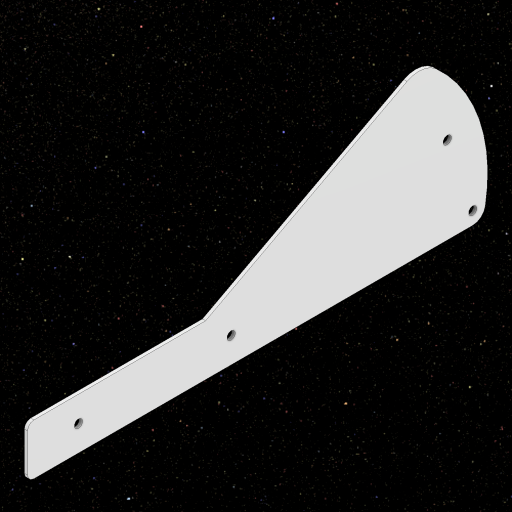
# Autodesk Inventor part: gusset_no_motor
Saved by Autodesk Inventor 2024 (Build 280153000, 153)
## iProperties
Created: 2024-02-12
Part Number: gusset_no_motor
Material: Acetal Resin, White
Document SubType Name: Modeling
Designer: Averey Ku
Density: 1.425 g/cm^3
Appearance: Smooth - White
Author: Averey Ku
Autodesk Inventor part; units mm, degrees
ref_plane "YZ Plane" through (0, 0, 0) normal (1, 0, 0) x (0, 1, 0)
ref_plane "XZ Plane" through (0, 0, 0) normal (0, 1, 0) x (-1, 0, 0)
ref_plane "XY Plane" through (0, 0, 0) normal (0, 0, 1) x (1, 0, 0)
sketch "main" plane through (0, 0, 0) normal (0, 0, 1) x (1, 0, 0)
  circle A0 centre (-31.9195, -99.4713) radius 2.0955
  arc A1 (-38.2695, -99.4713) -> (-33.0376, -105.722) centre (-31.9195, -99.4713) ccw
  arc A2 (-33.0376, -105.722) -> (38.5686, -81.1636) centre (-19.3218, -29.0418) ccw
  line L0 (40.3562, -66.7269) -> (-12.8695, 33.8787)
  line L1 (-12.8695, 33.8787) -> (-12.8695, 119.6037)
  line L2 (-16.0445, 122.7787) -> (-35.0945, 122.7787)
  line L3 (-38.2695, 119.6037) -> (-38.2695, -99.4713)
  arc A3 (38.5686, -81.1636) -> (40.3562, -66.7269) centre (29.1304, -72.6659) ccw
  circle A4 centre (-25.5695, 21.1787) radius 2.0955
  arc A5 (-12.8695, 119.6037) -> (-16.0445, 122.7787) centre (-16.0445, 119.6037) ccw
  circle A6 centre (5.0055, -86.7713) radius 2.0955
  circle A7 centre (-25.5695, 97.3787) radius 2.0955
  arc A8 (-35.0945, 122.7787) -> (-38.2695, 119.6037) centre (-35.0945, 119.6037) ccw
  point P0 (-9.1863, -18.3686)
  point P1 (44.2418, -74.0713)
  dimension "d0" = 4.191
  dimension "d1" = 12.7
  dimension "d3" = 4.191
  dimension "d4" = 3.175
  dimension "d5" = 4.191
  dimension "d17" = 4.191
  dimension "d18" = 3.175
  measures "d0" diameter of A0
  measures "d1" radius of A3
  measures "d3" diameter of A4
  measures "d4" radius of A5
  measures "d5" diameter of A6
  measures "d17" diameter of A7
  measures "d18" radius of A8
sketch "Sketch1" plane through (0, 0, 0) normal (1, 0, 0) x (0, 1, 0)
  circle A0 centre (-6.35, -209.55) radius 2.0955
  arc A1 (-12.7, -209.55) -> (-7.4681, -215.8008) centre (-6.35, -209.55) ccw
  arc A2 (-7.4681, -215.8008) -> (64.1381, -191.2423) centre (6.2477, -139.1205) ccw
  line L0 (65.9257, -176.8056) -> (12.7, -76.2)
  line L1 (12.7, -76.2) -> (12.7, 9.525)
  line L2 (9.525, 12.7) -> (-9.525, 12.7)
  line L3 (-12.7, 9.525) -> (-12.7, -209.55)
  arc A3 (64.1381, -191.2423) -> (65.9257, -176.8056) centre (54.7, -182.7446) ccw
  circle A4 centre (0, -88.9) radius 2.0955
  arc A5 (12.7, 9.525) -> (9.525, 12.7) centre (9.525, 9.525) ccw
  circle A6 centre (30.575, -196.85) radius 2.0955
  circle A7 centre (0, -12.7) radius 2.0955
  arc A8 (-9.525, 12.7) -> (-12.7, 9.525) centre (-9.525, 9.525) ccw
  point P0 (0, 0)
extrude "Extrusion1" add sketch "Sketch1" along normal blind 1.5875
body "Solid1"
